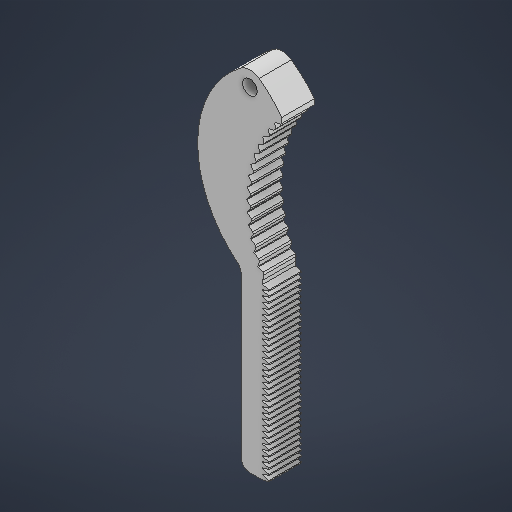
# Autodesk Inventor part: gripper part
Saved by Autodesk Inventor 2026.1 (Build 301233000, 233)
## iProperties
Created: 2025-10-10
Part Number: gripper part
Material: Generic
Document SubType Name: Modeling
Designer: shahn
Density: 1 g/cm^3
Appearance: Default
Author: shahn
Autodesk Inventor part; units mm, degrees
ref_plane "YZ Plane" through (0, 0, 0) normal (1, 0, 0) x (0, 1, 0)
ref_plane "XZ Plane" through (0, 0, 0) normal (0, 1, 0) x (-1, 0, 0)
ref_plane "XY Plane" through (0, 0, 0) normal (0, 0, 1) x (1, 0, 0)
sketch "Sketch1" plane through (0, 0, 0) normal (0, 0, 1) x (1, 0, 0)
  line L0 (23.6777, 0) -> (23.6777, 14.5214)
  line L1 (23.6777, 14.5214) -> (25.1266, 14.1331)
  line L2 (25.1266, 14.1331) -> (25.1266, 13.8831)
  line L3 (25.1266, 13.8831) -> (23.6777, 13.4949)
  line L4 (23.6777, 13.2946) -> (25.1266, 12.9063)
  line L5 (25.1266, 12.9063) -> (25.1266, 12.6563)
  line L6 (25.1266, 12.6563) -> (23.6777, 12.2681)
  line L7 (23.6777, 12.0677) -> (25.1266, 11.6795)
  line L8 (25.1266, 11.6795) -> (25.1266, 11.4295)
  line L9 (25.1266, 11.4295) -> (23.6777, 11.0413)
  line L10 (23.6777, 10.8409) -> (25.1266, 10.4527)
  line L11 (25.1266, 10.4527) -> (25.1266, 10.2027)
  line L12 (25.1266, 10.2027) -> (23.6777, 9.8145)
  line L13 (23.6777, 9.6141) -> (25.1266, 9.2259)
  line L14 (25.1266, 9.2259) -> (25.1266, 8.9759)
  line L15 (25.1266, 8.9759) -> (23.6777, 8.5877)
  line L16 (23.6777, 8.3873) -> (25.1266, 7.9991)
  line L17 (25.1266, 7.9991) -> (25.1266, 7.7491)
  line L18 (25.1266, 7.7491) -> (23.6777, 7.3609)
  line L19 (23.6777, 7.1605) -> (25.1266, 6.7723)
  line L20 (25.1266, 6.7723) -> (25.1266, 6.5223)
  line L21 (25.1266, 6.5223) -> (23.6777, 6.134)
  line L22 (23.6777, 5.9337) -> (25.1266, 5.5455)
  line L23 (25.1266, 5.5455) -> (25.1266, 5.2955)
  line L24 (25.1266, 5.2955) -> (23.6777, 4.9072)
  line L25 (23.6777, 4.7069) -> (25.1266, 4.3186)
  line L26 (25.1266, 4.3186) -> (25.1266, 4.0686)
  line L27 (25.1266, 4.0686) -> (23.6777, 3.6804)
  line L28 (23.6777, 3.4801) -> (25.1266, 3.0918)
  line L29 (25.1266, 3.0918) -> (25.1266, 2.8418)
  line L30 (25.1266, 2.8418) -> (23.6777, 2.4536)
  line L31 (23.6777, 2.2533) -> (25.1266, 1.865)
  line L32 (25.1266, 1.865) -> (25.1266, 1.615)
  line L33 (25.1266, 1.615) -> (23.6777, 1.2268)
  line L34 (23.6777, 1.0264) -> (25.1266, 0.6382)
  line L35 (25.1266, 0.6382) -> (25.1266, 0.3882)
  line L36 (25.1266, 0.3882) -> (23.6777, 0)
  line L37 (23.6777, 0) -> (18.6777, 0)
  line L38 (18.6777, 0) -> (18.6777, 40)
  line L39 (23.6777, 0) -> (23.6777, 40.0089)
  arc A0 (18.6122, 79.9999) -> (18.6777, 40) centre (33.6449, 60.0245) ccw
  arc A1 (23.6777, 40.0089) -> (22.8328, 79.9999) centre (8.2586, 59.6876) ccw
  arc A2 (22.8328, 79.9999) -> (18.6122, 79.9999) centre (20.7225, 77.1958) ccw
  line L40 (23.6777, 15.7544) -> (25.1266, 15.3661)
  line L41 (25.1266, 15.3661) -> (25.1266, 15.1161)
  line L42 (25.1266, 15.1161) -> (23.6777, 14.7279)
  line L43 (23.6777, 16.9874) -> (25.1266, 16.5991)
  line L44 (25.1266, 16.5991) -> (25.1266, 16.3491)
  line L45 (25.1266, 16.3491) -> (23.6777, 15.9609)
  line L46 (23.6777, 18.2204) -> (25.1266, 17.8321)
  line L47 (25.1266, 17.8321) -> (25.1266, 17.5821)
  line L48 (25.1266, 17.5821) -> (23.6777, 17.1939)
  line L49 (23.6777, 19.4534) -> (25.1266, 19.0651)
  line L50 (25.1266, 19.0651) -> (25.1266, 18.8151)
  line L51 (25.1266, 18.8151) -> (23.6777, 18.4269)
  line L52 (23.6777, 20.6864) -> (25.1266, 20.2981)
  line L53 (25.1266, 20.2981) -> (25.1266, 20.0481)
  line L54 (25.1266, 20.0481) -> (23.6777, 19.6599)
  line L55 (23.6777, 21.9194) -> (25.1266, 21.5311)
  line L56 (25.1266, 21.5311) -> (25.1266, 21.2811)
  line L57 (25.1266, 21.2811) -> (23.6777, 20.8929)
  line L58 (23.6777, 23.1524) -> (25.1266, 22.7641)
  line L59 (25.1266, 22.7641) -> (25.1266, 22.5141)
  line L60 (25.1266, 22.5141) -> (23.6777, 22.1259)
  line L61 (23.6777, 24.3854) -> (25.1266, 23.9971)
  line L62 (25.1266, 23.9971) -> (25.1266, 23.7471)
  line L63 (25.1266, 23.7471) -> (23.6777, 23.3589)
  line L64 (23.6777, 25.6184) -> (25.1266, 25.2301)
  line L65 (25.1266, 25.2301) -> (25.1266, 24.9801)
  line L66 (25.1266, 24.9801) -> (23.6777, 24.5919)
  line L67 (23.6777, 26.8514) -> (25.1266, 26.4631)
  line L68 (25.1266, 26.4631) -> (25.1266, 26.2131)
  line L69 (25.1266, 26.2131) -> (23.6777, 25.8249)
  line L70 (23.6777, 28.0844) -> (25.1266, 27.6961)
  line L71 (25.1266, 27.6961) -> (25.1266, 27.4461)
  line L72 (25.1266, 27.4461) -> (23.6777, 27.0579)
  line L73 (23.6777, 29.3174) -> (25.1266, 28.9291)
  line L74 (25.1266, 28.9291) -> (25.1266, 28.6791)
  line L75 (25.1266, 28.6791) -> (23.6777, 28.2909)
  line L76 (23.6777, 30.5504) -> (25.1266, 30.1621)
  line L77 (25.1266, 30.1621) -> (25.1266, 29.9121)
  line L78 (25.1266, 29.9121) -> (23.6777, 29.5239)
  line L79 (23.6777, 31.7834) -> (25.1266, 31.3951)
  line L80 (25.1266, 31.3951) -> (25.1266, 31.1451)
  line L81 (25.1266, 31.1451) -> (23.6777, 30.7569)
  line L82 (23.6777, 33.0164) -> (25.1266, 32.6281)
  line L83 (25.1266, 32.6281) -> (25.1266, 32.3781)
  line L84 (25.1266, 32.3781) -> (23.6777, 31.9899)
  line L85 (23.6777, 34.2494) -> (25.1266, 33.8611)
  line L86 (25.1266, 33.8611) -> (25.1266, 33.6111)
  line L87 (25.1266, 33.6111) -> (23.6777, 33.2229)
  line L88 (23.6777, 35.4824) -> (25.1266, 35.0941)
  line L89 (25.1266, 35.0941) -> (25.1266, 34.8441)
  line L90 (25.1266, 34.8441) -> (23.6777, 34.4559)
  line L91 (23.6777, 36.7154) -> (25.1266, 36.3271)
  line L92 (25.1266, 36.3271) -> (25.1266, 36.0771)
  line L93 (25.1266, 36.0771) -> (23.6777, 35.6889)
  line L94 (23.6777, 37.9484) -> (25.1266, 37.5601)
  line L95 (25.1266, 37.5601) -> (25.1266, 37.3101)
  line L96 (25.1266, 37.3101) -> (23.6777, 36.9219)
  line L97 (23.6777, 39.1814) -> (25.1266, 38.7931)
  line L98 (25.1266, 38.7931) -> (25.1266, 38.5431)
  line L99 (25.1266, 38.5431) -> (23.6777, 38.1549)
  point P0 (0, 0)
  point P1 (23.6777, 7.2607)
  point P2 (23.6777, 1.2268)
  point P3 (23.6777, 2.2533)
  point P4 (23.6777, 2.4536)
  point P5 (23.6777, 3.4801)
  point P6 (23.6777, 3.6804)
  point P7 (23.6777, 4.7069)
  point P8 (23.6777, 4.9072)
  point P9 (23.6777, 5.9337)
  point P10 (23.6777, 7.1605)
  point P11 (23.6777, 8.3873)
  point P12 (23.6777, 8.5877)
  point P13 (23.6777, 9.6141)
  point P14 (23.6777, 9.8145)
  point P15 (23.6777, 10.8409)
  point P16 (23.6777, 11.0413)
  point P17 (23.6777, 12.0677)
  point P18 (20.7225, 80.7053)
  point P19 (33.253, 60.2156)
  dimension "d8" = 23.6777
  dimension "d10" = 1.5
  dimension "d11" = 75
  dimension "d12" = 0.25
  dimension "d13" = 75
  dimension "d16" = 1.2268
  dimension "d38" = 5
  dimension "d39" = 40
  dimension "d40" = 40
  dimension "d41" = 25
  dimension "d42" = 40
  dimension "d43" = 25
  dimension "d44" = 0.2004
  dimension "d47" = 1.233
  dimension "d52" = 3.5095
  dimension "d53" = 40
  dimension "d54" = 59.6876
  dimension "d55" = 33.253
  dimension "d56" = 80.7053
  constraints: 196 end point, 124 vertical alignment, 62 parallel, 31 collinear, 8 point on circle, 3 centre point, 1 horizontal, 1 perpendicular, 1 tangent, 1 vertical, 8 other
  measures "d8" horizontal distance of point (0, 0) point (23.678, 7.261)
  measures "d10" distance of L1.start L1.end
  measures "d11" angle to the sketch y axis of L1
  measures "d12" distance of L1.end L2.end
  measures "d13" angle to the sketch y axis of L3
  measures "d16" distance of L1.start L4.start
  measures "d38" distance of L36.end L37.end
  measures "d39" distance of L37.end L38.end
  measures "d40" distance of L38.end A0.start
  measures "d41" radius of A0
  measures "d42" distance of A1.start A1.end
  measures "d43" radius of A1
  measures "d44" distance of L10.start L9.end
  measures "d47" distance of L1.start L40.start
  measures "d52" distance of point (20.722, 80.705) A2.centre
  measures "d53" vertical distance of point (0, 0) L38.end
  measures "d54" vertical distance of point (0, 0) A1.centre
  measures "d55" horizontal distance of point (33.253, 60.216) point (0, 0)
  measures "d56" vertical distance of point (0, 0) point (20.722, 80.705)
extrude "Extrusion5" add sketch "Sketch1" along normal blind 7.5
sketch "Sketch2" plane through (0, 0, 7.5) normal (0, 0, 1) x (1, 0, 0)
  arc A0 (23.6777, 40.0089) -> (22.8328, 79.9999) centre (8.2586, 59.6876) ccw projected
  line L0 (23.6777, 39.1814) -> (23.6777, 40.0089) projected
  arc A1 (28.1285, 74.8594) -> (23.6777, 40.0089) centre (50.026, 54.3534) ccw
  line L1 (23.6777, 40.0089) -> (23.9338, 41.1812)
  line L2 (23.9338, 41.1812) -> (23.7453, 41.6443)
  line L3 (23.7453, 41.6443) -> (22.6387, 42.1085)
  line L4 (22.7739, 43.8884) -> (21.71, 44.4435)
  line L5 (22.9229, 43.4111) -> (22.7739, 43.8884)
  line L6 (22.5696, 42.2643) -> (22.9229, 43.4111)
  line L7 (21.9937, 46.2058) -> (20.98, 46.8481)
  line L8 (22.1022, 45.7177) -> (21.9937, 46.2058)
  line L9 (21.6542, 44.6045) -> (22.1022, 45.7177)
  line L10 (21.4101, 48.5804) -> (20.4538, 49.3053)
  line L11 (21.4775, 48.085) -> (21.4101, 48.5804)
  line L12 (20.9378, 47.0132) -> (21.4775, 48.085)
  line L13 (21.0274, 50.9956) -> (20.1351, 51.7979)
  line L14 (21.053, 50.4962) -> (21.0274, 50.9956)
  line L15 (20.4256, 49.4733) -> (21.053, 50.4962)
  line L16 (20.8481, 53.4342) -> (20.0261, 54.3084)
  line L17 (20.8319, 52.9345) -> (20.8481, 53.4342)
  line L18 (20.121, 51.9677) -> (20.8319, 52.9345)
  line L19 (20.8735, 55.8794) -> (20.1275, 56.8193)
  line L20 (20.8155, 55.3827) -> (20.8735, 55.8794)
  line L21 (20.0263, 54.4788) -> (20.8155, 55.3827)
  line L22 (21.1035, 58.3138) -> (20.4388, 59.3129)
  line L23 (21.0042, 57.8238) -> (21.1035, 58.3138)
  line L24 (20.142, 56.9891) -> (21.0042, 57.8238)
  line L25 (21.5364, 60.7204) -> (20.9577, 61.7716)
  line L26 (21.3964, 60.2404) -> (21.5364, 60.7204)
  line L27 (20.4674, 59.4808) -> (21.3964, 60.2404)
  line L28 (22.1693, 63.0824) -> (21.6805, 64.1783)
  line L29 (21.9896, 62.6158) -> (22.1693, 63.0824)
  line L30 (21.0003, 61.9366) -> (21.9896, 62.6158)
  line L31 (22.9975, 65.3831) -> (22.6022, 66.5161)
  line L32 (22.7794, 64.9332) -> (22.9975, 65.3831)
  line L33 (21.7367, 64.3392) -> (22.7794, 64.9332)
  line L34 (24.0154, 67.6064) -> (23.7163, 68.7686)
  line L35 (23.7604, 67.1764) -> (24.0154, 67.6064)
  line L36 (22.6717, 66.6717) -> (23.7604, 67.1764)
  line L37 (25.2158, 69.7368) -> (25.015, 70.9199)
  line L38 (24.9257, 69.3295) -> (25.2158, 69.7368)
  line L39 (23.7986, 68.9178) -> (24.9257, 69.3295)
  line L40 (26.5903, 71.7592) -> (26.4892, 72.9549)
  line L41 (26.2671, 71.3777) -> (26.5903, 71.7592)
  line L42 (25.1095, 71.0616) -> (26.2671, 71.3777)
  line L43 (28.1292, 73.6595) -> (28.1285, 74.8595)
  line L44 (27.7753, 73.3063) -> (28.1292, 73.6595)
  line L45 (26.5952, 73.0883) -> (27.7753, 73.3063)
  arc A2 (22.8328, 79.9999) -> (18.6122, 79.9999) centre (20.7225, 77.1958) ccw projected
  point P0 (0, 0)
  point P1 (20.7225, 80.7053)
  point P2 (28.1285, 74.8594)
  dimension "d59" = 30
  dimension "d60" = 1.2
  dimension "d61" = 0.5
  dimension "d62" = 1.2
  dimension "d63" = 134.9
  dimension "d64" = 145.535
  dimension "d67" = 67.21
  dimension "d69" = 7.406
  constraints: 90 end point, 2 point on circle, 104 other
  measures "d60" distance of L0.end L1.end
  measures "d61" distance of L1.end L2.end
  measures "d62" distance of L2.end L3.end
  measures "d63" angle of L2 L3
  measures "d64" angle of L1 L2
  measures "d69" horizontal distance of point (20.722, 80.705) L43.end
extrude "Extrusion6" cut sketch "Sketch2" against normal blind 10 contours L1 L2 L3 A1 L6 L5 L4 L9 L8 L7 L12 L11 L10 L15 L14 L13 L18 L17 L16 L21 L20 L19 L24 L23 L22 L27 L26 L25 L30 L29 L28 L33 L32 L31 L36 L35 L34 L39 L38 L37 L42 L41 L40 L45 L44 L43 A0
fillet "Fillet3" radius 2 1 edges at (18.6777, 0, 3.75)
fillet "Fillet4" radius 2 1 edges at (18.6777, 40, 3.75)
sketch "Sketch3" plane through (0, 0, 7.5) normal (0, 0, 1) x (1, 0, 0)
  circle A0 centre (20.7225, 77.1958) radius 1.7
  arc A1 (22.8328, 79.9999) -> (18.6122, 79.9999) centre (20.7225, 77.1958) ccw projected
  point P0 (0, 0)
  dimension "d74" = 3.4
  constraints: 1 centre point, 1 concentric
  measures "d74" diameter of A0
extrude "Extrusion7" cut sketch "Sketch3" against normal blind 10
body "Solid5"
